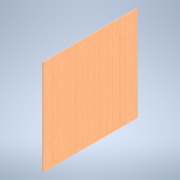
# Autodesk Inventor part: front_cover
Saved by Autodesk Inventor 2020 (Build 240168000, 168)
## iProperties
Created: 2020-05-03
Part Number: front_cover
Material: Generic
Document SubType Name: Modeling
Designer: galaxy
Density: 1 g/cm^3
Appearance: Default
Author: galaxy
Autodesk Inventor part; units mm, degrees
ref_plane "YZ Plane" through (0, 0, 0) normal (1, 0, 0) x (0, 1, 0)
ref_plane "XZ Plane" through (0, 0, 0) normal (0, 1, 0) x (-1, 0, 0)
ref_plane "XY Plane" through (0, 0, 0) normal (0, 0, 1) x (1, 0, 0)
sketch "Sketch1" plane through (0, 0, 0) normal (1, 0, 0) x (0, 1, 0)
  line L0 (179, 179) -> (-179, 179)
  line L1 (-179, 179) -> (-179, -179)
  line L2 (-179, -179) -> (179, -179)
  line L3 (179, -179) -> (179, 179)
  line L4 (179, 179) -> (-179, -179) construction
  line L5 (-179, 179) -> (179, -179) construction
  point P0 (0, 0)
  dimension "d0" = 358
  dimension "d1" = 358
  constraints: 12 end point, 2 midpoint, 2 parallel, 1 horizontal, 1 perpendicular
  measures "d0" distance of L2.end L1.end
  measures "d1" distance of L1.end L0.end
extrude "Extrusion1" add sketch "Sketch1" along normal blind 3
sketch "Sketch2" plane through (3, 0, 0) normal (1, 0, 0) x (0, 0, -1)
  circle A0 centre (-171, 165) radius 1.875
  circle A1 centre (-171, 139.2) radius 1.875
  circle A2 centre (-171, 113.4) radius 1.875
  line L0 (179, 179) -> (-179, 179) projected
  line L1 (-179, 179) -> (-179, -179) projected
  point P0 (0, 0)
  dimension "d4" = 3.75
  dimension "d5" = 3.75
  dimension "d6" = 3.75
  dimension "d7" = 14
  dimension "d8" = 25.8
  dimension "d9" = 25.8
  dimension "d10" = 8
  constraints: 3 centre point
  measures "d4" diameter of A0
  measures "d5" diameter of A1
  measures "d6" diameter of A2
  measures "d7" distance from line of L0 A0.centre
  measures "d8" distance of A0.centre A1.centre
  measures "d9" distance of A1.centre A2.centre
  measures "d10" distance from line of L1 A0.centre
extrude "Extrusion2" cut sketch "Sketch2" against normal blind 3
mirror "Mirror1" about plane through (0, 0, 0) normal (0, 1, 0) of "Extrusion2"
sketch "Sketch3" plane through (3, 0, 0) normal (1, 0, 0) x (0, 0, -1)
  line L0 (-179, 179) -> (-176.5, 179)
  line L1 (179, 179) -> (-179, 179) projected
  line L2 (-176.5, 179) -> (-176.5, -179)
  line L3 (-179, -179) -> (179, -179) projected
  line L4 (-176.5, -179) -> (-179, -179)
  line L5 (-179, -179) -> (-179, 179)
  point P0 (0, 0)
  dimension "d13" = 2.5
  dimension "d14" = 90
  constraints: 8 end point, 2 point on line, 1 collinear, 1 perpendicular
  measures "d13" distance of L0.start L0.end
  measures "d14" angle of L0 L2
extrude "Extrusion3" cut sketch "Sketch3" against normal blind 3
body "Solid1"
